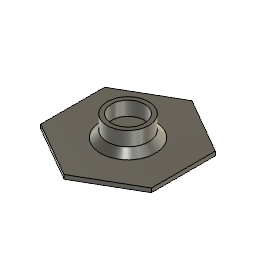
WiFi_Controlled_Desk_Lamp_Twisted_Top (Autodesk Fusion 360 design; units mm, degrees)
part number: 2026-05-21-09-09-44-045
Autodesk Fusion 360 part; units mm, degrees
sketch "Sketch1" plane through (0, 0, 0) normal (0, 0, 1) x (1, 0, 0)
  line L0 (33.4251, -19.298) -> (33.4251, 19.298)
  line L1 (33.4251, 19.298) -> (0, 38.596)
  line L2 (0, 38.596) -> (-33.4251, 19.298)
  line L3 (-33.4251, 19.298) -> (-33.4251, -19.298)
  line L4 (-33.4251, -19.298) -> (0, -38.596)
  line L5 (0, -38.596) -> (33.4251, -19.298)
  dimension "d1" = 38.596
  constraint vertical origin L1.end
  measures "d1" distance of L1.end origin
extrude "Extrude1" add sketch "Sketch1" along normal blind 2.5
sketch "Sketch2" plane through (0, 0, 2.5) normal (0, 0, 1) x (-1, 0, 0)
  line L0 (0, 38.596) -> (-33.4251, 19.298)
  line L1 (-33.4251, 19.298) -> (-33.4251, -19.298)
  line L2 (-33.4251, -19.298) -> (0, -38.596)
  line L3 (0, -38.596) -> (33.4251, -19.298)
  line L4 (33.4251, -19.298) -> (33.4251, 19.298)
  line L5 (33.4251, 19.298) -> (0, 38.596)
  circle A0 centre (0, 0) radius 16.5
  dimension "d4" = 33
  constraint coincident A0.centre origin
  measures "d4" diameter of A0
extrude "Extrude2" add sketch "Sketch2" along normal blind 4 draft -45 contours A0
sketch "Sketch3" plane through (0, 0, 6.5) normal (0, 0, 1) x (-1, 0, 0)
  circle A0 centre (0, 0) radius 12.5
  circle A1 centre (0, 0) radius 10
  dimension "d7" = 20
  constraint coincident A0.centre A1.centre
  measures "d7" diameter of A1
extrude "Extrude3" add sketch "Sketch3" along normal blind 8.5
